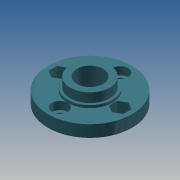
# Autodesk Inventor part: bearing seat 2
Saved by Autodesk Inventor 2013 (Build 170138000, 138)
## iProperties
Created: 2017-04-04
Part Number: bearing seat 2
Material: Generic
Document SubType Name: Modeling
Designer: employee
Density: 1 g/cm^3
Author: employee
Autodesk Inventor part; units mm, degrees
ref_plane "YZ Plane" through (0, 0, 0) normal (1, 0, 0) x (0, 1, 0)
ref_plane "XZ Plane" through (0, 0, 0) normal (0, 1, 0) x (-1, 0, 0)
ref_plane "XY Plane" through (0, 0, 0) normal (0, 0, 1) x (1, 0, 0)
sketch "Sketch1" plane through (0, 0, 0) normal (0, 0, 1) x (1, 0, 0)
  circle A0 centre (0, 0) radius 16
  dimension "d0" = 32
  constraints: 1 centre point, 1 coincident
  measures "d0" diameter of A0
extrude "Extrusion1" add sketch "Sketch1" along normal blind 4.5
sketch "Sketch2" plane through (0, 0, 4.5) normal (0, 0, 1) x (1, 0, 0)
  circle A0 centre (0, 0) radius 16 projected
  circle A1 centre (0, 0) radius 8.5
  dimension "d5" = 17
  constraints: 1 centre point, 1 coincident
  measures "d5" diameter of A1
extrude "Extrusion2" add sketch "Sketch2" along normal blind 1 contours A1
sketch "Sketch3" plane through (0, 0, 5.5) normal (0, 0, 1) x (1, 0, 0)
  circle A0 centre (0, 0) radius 8.5 projected
  circle A1 centre (0, 0) radius 7.5
  dimension "d10" = 15
  constraints: 1 centre point, 1 coincident
  measures "d10" diameter of A1
extrude "Extrusion3" cut sketch "Sketch3" against normal through all contours A1
sketch "Sketch4" plane through (0, 0, 4.5) normal (0, 0, 1) x (1, 0, 0)
  circle A0 centre (0, 0) radius 8.5 projected
  circle A1 centre (0, 11.5) radius 1.75
  circle A2 centre (0, 11.5) radius 3
  dimension "d15" = 11.5
  dimension "d16" = 3.5
  dimension "d41" = 6
  constraints: 2 centre point, 1 coincident, 1 vertical alignment
  measures "d15" distance of A0.centre A1.centre
  measures "d16" diameter of A1
  measures "d41" diameter of A2
extrude "Extrusion4" cut sketch "Sketch4" against normal through all contours A1
pattern_circular "Circular Pattern1" count 4 over 360 about axis through (0, 0, 0) along (0, 0, 1) of "Extrusion4"
sketch "Sketch5" plane through (0, 0, 4.5) normal (0, 0, 1) x (1, 0, 0)
  circle A0 centre (0, 11.5) radius 1.75 projected
  circle A1 centre (0, 0) radius 8.5 projected
  arc A2 (0, 8.5) -> (0, 8.5) centre (0, 11.5) ccw
  circle A3 centre (0, 11.5) radius 3
  dimension "d22" = 6
  dimension "d40" = 6
  constraints: 4 point on circle, 2 centre point, 2 coincident
  measures "d22" diameter of A2
  measures "d40" diameter of A3
extrude "Extrusion5" cut sketch "Sketch5" against normal blind 3
sketch "Sketch6" plane through (0, 0, 4.5) normal (0, 0, 1) x (1, 0, 0)
  circle A0 centre (-11.5, 0) radius 1.75 projected
  line L0 (-11.5, 3.1754) -> (-8.75, 1.5877)
  line L1 (-8.75, 1.5877) -> (-8.75, -1.5877)
  line L2 (-8.75, -1.5877) -> (-11.5, -3.1754)
  line L3 (-11.5, -3.1754) -> (-14.25, -1.5877)
  line L4 (-14.25, -1.5877) -> (-14.25, 1.5877)
  line L5 (-14.25, 1.5877) -> (-11.5, 3.1754)
  dimension "d28" = 5.5
  constraints: 12 end point, 1 coincident, 1 vertical, 13 other
  measures "d28" distance between parallel lines of L4 L1
extrude "Extrusion6" cut sketch "Sketch6" against normal blind 4
pattern_circular "Circular Pattern2" count 2 over 360 about axis through (0, 0, 0) along (0, 0, 1) of "Extrusion6", "Extrusion5"
sketch "Sketch7" plane through (0, 0, 0) normal (0, 0, -1) x (-1, 0, 0)
  circle A0 centre (0, 0) radius 7.5 projected
  circle A1 centre (0, 0) radius 16 projected
  circle A2 centre (0, 0) radius 5
  dimension "d34" = 10
  constraints: 1 centre point, 1 coincident
  measures "d34" diameter of A2
extrude "Extrusion7" add sketch "Sketch7" against normal blind 9 contours A0
body "Solid1"
